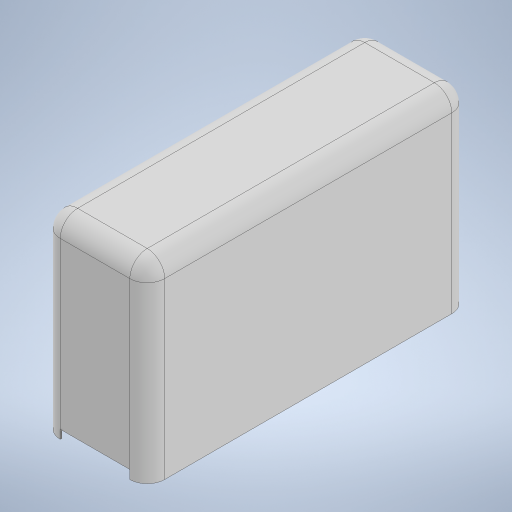
# Autodesk Inventor part: Top_Case
Saved by Autodesk Inventor 2024 (Build 280153000, 153)
## iProperties
Created: 2023-11-21
Part Number: Top_Case
Material: Generic
Document SubType Name: Modeling
Designer: renan
Density: 1 g/cm^3
Appearance: Default
Author: renan
Autodesk Inventor part; units mm, degrees
ref_plane "YZ Plane" through (0, 0, 0) normal (1, 0, 0) x (0, 1, 0)
ref_plane "XZ Plane" through (0, 0, 0) normal (0, 1, 0) x (-1, 0, 0)
ref_plane "XY Plane" through (0, 0, 0) normal (0, 0, 1) x (1, 0, 0)
sketch "Sketch1" plane through (0, 0, 0) normal (0, 1, 0) x (-1, 0, 0)
  line L0 (0, 0) -> (-12, 0)
  line L1 (-12, 0) -> (-12, -37)
  line L2 (-12, -37) -> (0, -37)
  line L3 (0, -37) -> (0, 0)
  dimension "d0" = 12
  dimension "d1" = 37
  constraints: 8 end point, 2 parallel, 1 horizontal, 1 perpendicular
  measures "d0" distance of L1.end L2.end
  measures "d1" distance of L0.end L1.end
extrude "Extrusion1" add sketch "Sketch1" along normal blind 22
fillet "Fillet1" radius 2 8 edges at (6, 22, -37) (0, 22, -18.5) (12, 22, -18.5) (6, 22, 0) (0, 11, 0) (0, 11, -37) (12, 11, -37) (12, 11, 0)
shell "Shell1" thickness 0.2 removed faces 1 at (8, 0, -13)
sketch "Sketch2" plane through (2, 0, 0) normal (0, 0, 1) x (1, 0, 0)
  line L0 (8, 0) -> (0, 0) projected
  line L1 (8, 0) -> (8, 20) projected
  line L2 (0, 0) -> (8, 0)
  line L3 (8, 0) -> (8, 1)
  line L4 (8, 1) -> (0, 1)
  line L5 (0, 1) -> (0, 0)
  point P0 (-2, 0)
  dimension "d6" = 1
  constraints: 8 end point, 2 parallel, 1 horizontal, 1 perpendicular, 1 point on line
  measures "d6" distance of L4.end L0.end
extrude "Extrusion2" cut sketch "Sketch2" against normal blind 22
body "Solid1"
